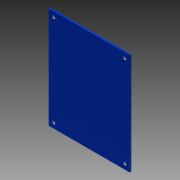
# Autodesk Inventor part: Platine_MCU
Saved by Autodesk Inventor 2015 (Build 190159000, 159)
## iProperties
Created: 2018-03-07
Part Number: Platine_MCU
Material: Generisch
Document SubType Name: Modeling
Designer: wepet
Density: 1 g/cm^3
Appearance: Vorgabe
Author: wepet
Autodesk Inventor part; units mm, degrees
ref_plane "YZ Plane" through (0, 0, 0) normal (1, 0, 0) x (0, 1, 0)
ref_plane "XZ Plane" through (0, 0, 0) normal (0, 1, 0) x (-1, 0, 0)
ref_plane "XY Plane" through (0, 0, 0) normal (0, 0, 1) x (1, 0, 0)
sketch "Skizze1" plane through (0, 0, 0) normal (0, 1, 0) x (-1, 0, 0)
  line L0 (40, 50) -> (-40, 50)
  line L1 (-40, 50) -> (-40, -50)
  line L2 (-40, -50) -> (40, -50)
  line L3 (40, -50) -> (40, 50)
  line L4 (0, 0) -> (0, -50) construction
  line L5 (0, 0) -> (40, 0) construction
  line L6 (35, 45) -> (-35, 45) construction
  line L7 (-35, 45) -> (-35, -45) construction
  line L8 (-35, -45) -> (35, -45) construction
  line L9 (35, -45) -> (35, 45) construction
  circle A0 centre (35, 45) radius 1.5
  circle A1 centre (-35, 45) radius 1.5
  circle A2 centre (-35, -45) radius 1.5
  circle A3 centre (35, -45) radius 1.5
  point P0 (35, 0)
  point P1 (0, -45)
  dimension "d0" = 100
  dimension "d1" = 80
  dimension "d2" = 5
  dimension "d3" = 5
  dimension "d4" = 3
  dimension "d5" = 3
  dimension "d6" = 3
  dimension "d7" = 3
  constraints: 20 end point, 5 midpoint, 4 centre point, 4 coincident, 4 parallel, 4 perpendicular, 3 point on line, 2 horizontal
  measures "d0" distance between parallel lines of L2 L0
  measures "d1" distance of L1.end L2.end
  measures "d2" distance between parallel lines of L2 L8
  measures "d3" distance between parallel lines of L3 L9
  measures "d4" diameter of A0
  measures "d5" diameter of A1
  measures "d6" diameter of A2
  measures "d7" diameter of A3
extrude "Extrusion1" add sketch "Skizze1" along normal blind 1.6
